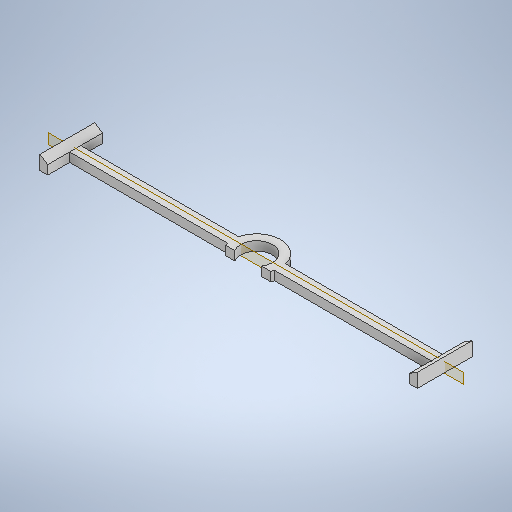
# Autodesk Inventor part: 2024_08_23_Holder_GC_vial
Saved by Autodesk Inventor 2025.1 (Build 291241000, 241)
## iProperties
Created: 2024-08-23
Part Number: 2024_08_23_Holder_GC_vial
Material: Generisch
Document SubType Name: Modeling
Designer: to86hug
Density: 1 g/cm^3
Appearance: Vorgabe
Author: to86hug
Autodesk Inventor part; units mm, degrees
ref_plane "YZ Plane" through (0, 0, 0) normal (1, 0, 0) x (0, 1, 0)
ref_plane "XZ Plane" through (0, 0, 0) normal (0, 1, 0) x (-1, 0, 0)
ref_plane "XY Plane" through (0, 0, 0) normal (0, 0, 1) x (1, 0, 0)
sketch "Skizze1" plane through (0, 0, 0) normal (0, 0, 1) x (1, 0, 0)
  line L0 (-68.016, 1.808) -> (67.584, 1.808)
  line L1 (67.584, 1.808) -> (67.584, -2.192)
  line L2 (67.584, -2.192) -> (-68.016, -2.192)
  line L3 (-68.016, -2.192) -> (-68.016, 1.808)
  line L4 (-68.016, 1.808) -> (67.584, -2.192) construction
  line L5 (67.584, 1.808) -> (-68.016, -2.192) construction
  point P0 (0, 0)
  point P1 (-0.216, -0.192)
  point P2 (-0.216, -0.192)
  dimension "d0" = 135.6
  dimension "d1" = 4
  constraints: 12 end point, 2 midpoint, 2 parallel, 1 horizontal, 1 perpendicular
  measures "d0" distance of L0.start L0.end
  measures "d1" distance of L0.end L1.end
extrude "Extrusion1" add sketch "Skizze1" along normal mid plane 3.25
ref_plane "Arbeitsebene1" through (-68.016, -0.192, 1.625) normal (0, -1, 0) x (1, 0, 0)
sketch "Skizze2" plane through (-68.016, -0.192, 1.625) normal (0, -1, 0) x (1, 0, 0)
  line L0 (0, -3.25) -> (0, 0) projected
  line L1 (0, -3.25) -> (135.6, -3.25) projected
  line L2 (0, 0) -> (2.85, 0)
  line L3 (2.85, 0) -> (2.85, -3.25)
  line L4 (2.85, -3.25) -> (0, -3.25)
  line L5 (0, -3.25) -> (0, 0)
  line L6 (0, 0) -> (0, 1.75)
  line L7 (0, 1.75) -> (2.85, 0)
  line L8 (135.6, -3.25) -> (135.6, 0) projected
  line L9 (135.6, 0) -> (132.75, 0)
  line L10 (132.75, 0) -> (132.75, -3.25)
  line L11 (132.75, -3.25) -> (135.6, -3.25)
  line L12 (135.6, -3.25) -> (135.6, 0)
  line L13 (135.6, 0) -> (135.6, 1.75)
  line L14 (135.6, 1.75) -> (132.75, 0)
  point P0 (68.016, -1.625)
  dimension "d4" = 2.85
  dimension "d5" = 1.75
  dimension "d6" = 2.85
  constraints: 24 end point, 4 parallel, 2 horizontal, 2 perpendicular, 2 point on line, 2 vertical
  measures "d4" distance of L3.end L4.end
  measures "d5" distance of L0.end L6.end
  measures "d6" distance of L11.end L10.end
extrude "Extrusion2" add sketch "Skizze2" along normal mid plane 19.7
sketch "Skizze3" plane through (0, 0, 1.625) normal (0, 0, 1) x (1, 0, 0)
  circle A0 centre (0, 0) radius 7.575
  dimension "d9" = 15.15
  constraints: 1 centre point, 1 coincident
  measures "d9" diameter of A0
extrude "Extrusion3" cut sketch "Skizze3" against normal through all
sketch "Skizze4" plane through (0, 0, -1.625) normal (0, 0, -1) x (-1, 0, 0)
  circle A0 centre (-0.0041, -0.1983) radius 8.65
  circle A1 centre (-0.0041, -0.1983) radius 5.65
  line L0 (10.587, -3.1983) -> (-10.6177, -3.1983)
  point P0 (-0.0041, -0.1983)
  point P1 (-8.1172, -3.1983)
  point P2 (-4.7918, -3.1983)
  point P3 (4.7837, -3.1983)
  point P4 (8.109, -3.1983)
  dimension "d27" = 11.3
  dimension "d28" = 17.3
  dimension "d29" = 3
  constraints: 2 centre point, 2 end point, 1 coincident
  measures "d27" diameter of A1
  measures "d28" diameter of A0
  measures "d29" distance from line of A1.centre L0
extrude "Extrusion4" add sketch "Skizze4" against normal blind 3.25 contours A0 L0 A1 picked at (7.4994, 0.9742)
equation "\"d28\" = d30"
equation "\"d30\" = 17.3"
